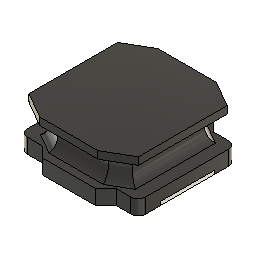
lqh44pn220mprl v4 (Autodesk Fusion 360 design; units mm, degrees)
Autodesk Fusion 360 part; units mm, degrees
note: some values were not read from the file. Set by a fixed rule: which sketch regions a step uses.
sketch "Sketch1" plane through (0, 0, 0) normal (0, 0, 1) x (1, 0, 0)
  line L0 (-2, 1.4) -> (-2, -1.4)
  line L1 (-1.75, -1.65) -> (-1.25, -1.65)
  line L2 (-1.25, -1.65) -> (-0.9, -2)
  line L3 (-0.9, -2) -> (0.9, -2)
  line L4 (0.9, -2) -> (1.25, -1.65)
  line L5 (1.25, -1.65) -> (1.75, -1.65)
  line L6 (2, -1.4) -> (2, 1.4)
  line L7 (1.75, 1.65) -> (1.25, 1.65)
  line L8 (1.25, 1.65) -> (0.9, 2)
  line L9 (0.9, 2) -> (-0.9, 2)
  line L10 (-0.9, 2) -> (-1.25, 1.65)
  line L11 (-1.25, 1.65) -> (-1.75, 1.65)
  line L12 (-1.25, 1.65) -> (1.25, 1.65) construction
  line L13 (1.25, -1.65) -> (-1.25, -1.65) construction
  line L14 (-0.9, 2) -> (-0.9, -2) construction
  line L15 (0.9, 2) -> (0.9, -2) construction
  line L16 (-0.9, 1.65) -> (0.9, -1.65) construction
  arc A0 (-1.75, 1.65) -> (-2, 1.4) centre (-1.75, 1.4) ccw
  arc A1 (-2, -1.4) -> (-1.75, -1.65) centre (-1.75, -1.4) ccw
  arc A2 (1.75, -1.65) -> (2, -1.4) centre (1.75, -1.4) ccw
  arc A3 (2, 1.4) -> (1.75, 1.65) centre (1.75, 1.4) ccw
  point P0 (-2, 1.65)
  point P1 (-2, -1.65)
  dimension "d1" = 3.3
  dimension "d2" = 4
  dimension "d3" = 1.8
  dimension "d4" = 45
  dimension "d5" = 45
  dimension "d6" = 45
  dimension "d7" = 45
  dimension "d8" = 4
  dimension "d9" = 0.25
  constraint vertical L0
  constraint horizontal L11
  constraint horizontal L1
  constraint horizontal L9
  constraint horizontal L3
  constraint vertical L6
  constraint horizontal L5
  constraint horizontal L7
  constraint horizontal L12
  constraint horizontal L13
  constraint vertical L15
  constraint vertical L14
  constraint equal L12 L13
  constraint coincident L14 L16.start
  constraint coincident L12 L16.start
  constraint coincident L15 L16.end
  constraint coincident L13 L16.end
  constraint midpoint origin L16
  constraint coincident P0 L0
  constraint coincident P0 L11
  constraint tangent L0 A0
  constraint tangent L11 A0
  constraint coincident P1 L0
  constraint coincident P1 L1
  constraint tangent L0 A1
  constraint tangent L1 A1
  constraint equal A0 A1
  constraint tangent L5 A2
  constraint tangent L6 A2
  constraint equal A0 A2
  constraint tangent L6 A3
  constraint tangent L7 A3
  constraint equal A0 A3
  constraint equal L7 L11
  measures "d1" distance of P0 P1
  measures "d2" distance of L0 L6
  measures "d3" distance of L2.end L3.end
  measures "d4" angle of L10 L12
  measures "d5" angle of L8 L12
  measures "d6" angle of L2 L13
  measures "d7" angle of L4 L13
  measures "d8" distance of L3 L9
  measures "d9" radius of A0
extrude "Extrude1" add sketch "Sketch1" along normal blind 0.5 makes body 1
ref_plane "WorkPlane1" through (0, 0, 1.65) normal (0, 0, 1) x (1, 0, 0)
sketch "Sketch2" plane through (0, 0, 1.65) normal (0, 0, 1) x (1, 0, 0)
  line L0 (1.85, -1.5) -> (-1.85, -1.5) construction
  line L1 (-1.85, -1.5) -> (-1.85, 1.5)
  line L2 (-1.85, 1.5) -> (1.85, 1.5) construction
  line L3 (1.85, 1.5) -> (1.85, -1.5)
  line L4 (-1.85, 1.5) -> (-0.984, 2)
  line L5 (-0.984, 2) -> (0.984, 2)
  line L6 (0.984, 2) -> (1.85, 1.5)
  line L7 (1.85, -1.5) -> (0.984, -2)
  line L8 (0.984, -2) -> (-0.984, -2)
  line L9 (-0.984, -2) -> (-1.85, -1.5)
  line L10 (-0.984, -2) -> (-0.984, 2) construction
  line L11 (0.984, 2) -> (0.984, -2) construction
  line L12 (-0.984, 1.5) -> (0.984, -1.5) construction
  dimension "d13" = 3.7
  dimension "d14" = 4
  dimension "d15" = 60
  dimension "d16" = 60
  dimension "d17" = 60
  dimension "d18" = 0.5
  constraint horizontal L0
  constraint vertical L1
  constraint horizontal L2
  constraint vertical L3
  constraint horizontal L5
  constraint horizontal L8
  constraint vertical L10
  constraint vertical L11
  constraint coincident L2 L12.start
  constraint coincident L10 L12.start
  constraint coincident L11 L12.end
  constraint coincident L0 L12.end
  constraint midpoint origin L12
  measures "d13" distance of L1.end L2.end
  measures "d14" distance of L4.end L8.end
  measures "d15" angle of L4 L10
  measures "d16" angle of L6 L11
  measures "d17" angle of L9 L10
  measures "d18" distance of L4.end L12.start
extrude "Extrude3" add sketch "Sketch2" against normal blind 1.15 bodies 1
ref_plane "WorkPlane4" through (0, 0, 0.825) normal (0, 0, 1) x (1, 0, 0)
sketch "Sketch6" plane through (0, 0, 0.825) normal (0, 0, 1) x (1, 0, 0)
  line L0 (-0.984, -2) -> (0.984, -2)
  line L1 (0.984, -2) -> (1.85, -1.5)
  line L2 (1.85, -1.5) -> (1.85, 1.5)
  line L3 (1.85, 1.5) -> (0.984, 2)
  line L4 (0.984, 2) -> (-0.984, 2)
  line L5 (-0.984, 2) -> (-1.85, 1.5)
  line L6 (-1.85, 1.5) -> (-1.85, -1.5)
  line L7 (-1.85, -1.5) -> (-0.984, -2)
ref_plane "WorkPlane5" through (0, 0, 1.075) normal (-1, 0, 0) x (0, 1, 0)
sketch "Sketch7" plane through (0, 0, 1.075) normal (-1, 0, 0) x (0, 1, 0)
  line L0 (2, -0.575) -> (1.5, -0.575)
  line L1 (2, -0.575) -> (2, 0.575)
  line L2 (2, -0.325) -> (1.5, -0.325) construction
  arc A0 (1.75, 0.575) -> (2, -0.325) centre (2, 0.1597) ccw
  line L3 (2, -0.325) -> (2, 0.575)
  line L4 (2, 0.575) -> (1.75, 0.575)
  dimension "d35" = 0.25
  dimension "d42" = 0.25
  constraint coincident L1 L2.start
  constraint perpendicular L1 L2
  constraint equal L0 L2
  constraint coincident L1 L3.end
  constraint coincident L1.end L3.end
  constraint coincident L1 A0.centre
  constraint perpendicular L3 L4
  measures "d35" distance of L0.start L2.start
  measures "d42" distance of L1.end A0.start
sweep "Sweep2" cut profiles "Sketch7" path "Sketch6" along L5 L6 L7 L0 L1 L2 L3 L4 section 1 bodies 1
sketch "Sketch8" plane through (0, 0, 0) normal (0, 0, 1) x (1, 0, 0)
  line L0 (-2, -1.65) -> (-0.9, -1.65) construction
  line L1 (-0.9, -1.65) -> (-0.9, 1.65)
  line L2 (-0.9, 1.65) -> (-2, 1.65) construction
  line L3 (-2, 1.65) -> (-2, -1.65) construction
  line L4 (-0.9, -1.65) -> (-1.05, -1.65)
  line L5 (-1.05, -1.2) -> (-1.85, -1.2)
  line L6 (-1.85, -1.2) -> (-1.85, -0.9094)
  line L7 (-1.85, -0.9094) -> (-2, -0.9094)
  line L8 (-2, 0.9094) -> (-1.85, 0.9094)
  line L9 (-1.85, 0.9094) -> (-1.85, 1.2)
  line L10 (-1.85, 1.2) -> (-1.05, 1.2)
  line L11 (-1.05, 1.2) -> (-1.05, 1.65)
  line L12 (-1.05, -1.65) -> (-1.05, -1.2)
  line L13 (-1.05, 1.65) -> (-0.9, 1.65)
  line L14 (-1.85, -0.9094) -> (-1.85, 0.9094) construction
  line L15 (-1.05, -1.2) -> (-1.05, 1.2) construction
  line L16 (-1.85, 0) -> (-0.9, 0) construction
  line L17 (-0.9, 0) -> (0, 0) construction
  line L18 (-2, -0.9094) -> (-2, 0.9094)
  line L19 (-2, 1.4) -> (-2, -1.4) construction
  dimension "d43" = 3.3
  dimension "d44" = 2.4
  dimension "d45" = 1.1
  dimension "d46" = 0.8
  constraint horizontal L0
  constraint vertical L1
  constraint horizontal L2
  constraint vertical L3
  constraint coincident L0 L4.end
  constraint perpendicular L1 L5
  constraint perpendicular L5 L6
  constraint coincident L3 L7.end
  constraint perpendicular L3 L7
  constraint coincident L3 L8.start
  constraint perpendicular L3 L8
  constraint perpendicular L2 L9
  constraint perpendicular L3 L10
  constraint coincident L2 L11.end
  constraint perpendicular L2 L11
  constraint perpendicular L5 L12
  constraint perpendicular L8 L14
  constraint vertical L15
  constraint equal L4 L7
  constraint midpoint L14 L16.start
  constraint midpoint L1 L16.end
  constraint symmetric L5 L10 L16
  constraint horizontal L17
  constraint coincident L17.end origin
  constraint coincident L3 L19.end
  measures "d43" distance of L0.end L1.end
  measures "d44" distance of L5.start L10.end
  measures "d45" distance of L1.end L2.end
  measures "d46" distance of L5.start L5.end
extrude "Extrude4" add sketch "Sketch8" along normal blind 0.12 separate body makes body 2
mirror "Mirror1" about plane through (0, 0, 0) normal (1, 0, 0) of bodies 2 makes body 3
combine "Combine1" operation cut target body 1 tool bodies 2 3 keep tools
